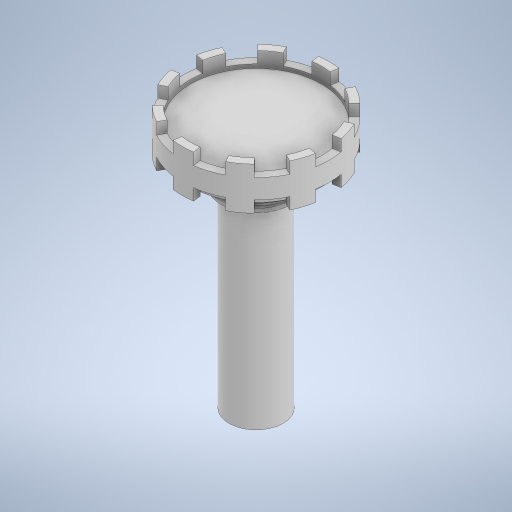
# Autodesk Inventor part: 另屋1 base
Saved by Autodesk Inventor 2024 (Build 280153000, 153)
## iProperties
Created: 2024-05-24
Part Number: 另屋1 base
Material: 一般
Document SubType Name: Modeling
Designer: User
Density: 1 g/cm^3
Appearance: 預設
Author: User
Autodesk Inventor part; units mm, degrees
ref_plane "YZ Plane" through (0, 0, 0) normal (1, 0, 0) x (0, 1, 0)
ref_plane "XZ Plane" through (0, 0, 0) normal (0, 1, 0) x (-1, 0, 0)
sketch "草圖1" plane through (0, 0, 0) normal (0, 1, 0) x (-1, 0, 0)
  circle A0 centre (0, 0) radius 19
  circle A1 centre (0, 0) radius 17
  dimension "d0" = 38
  dimension "d1" = 34
  constraints: 2 centre point, 2 coincident
  measures "d0" diameter of A0
  measures "d1" diameter of A1
extrude "擠出1" add sketch "草圖1" along normal blind 4 contours A1
extrude "擠出2" add sketch "草圖1" along normal blind 5
sketch "草圖2" plane through (0, 5, 0) normal (0, 1, 0) x (1, 0, 0)
  circle A0 centre (0, 0) radius 19
  circle A1 centre (0, 0) radius 17
  line L0 (0, 0) -> (2.6443, 18.8151)
  line L1 (0, 0) -> (-2.6443, 18.8151)
  line L2 (0, 0) -> (0, 13.9277)
  line L3 (0, 0) -> (-8.92, 16.776)
  line L4 (0, 0) -> (-13.1985, 13.6675)
  line L5 (0, 0) -> (-17.0771, 8.3291)
  line L6 (0, 0) -> (-18.7113, 3.2993)
  line L7 (0, 0) -> (-18.7113, -3.2993)
  line L8 (0, 0) -> (-17.0771, -8.3291)
  line L9 (0, 0) -> (-13.1985, -13.6675)
  line L10 (0, 0) -> (-8.92, -16.776)
  line L11 (0, 0) -> (-2.6443, -18.8151)
  line L12 (0, 0) -> (2.6443, -18.8151)
  line L13 (0, 0) -> (8.92, -16.776)
  line L14 (0, 0) -> (13.1985, -13.6675)
  line L15 (0, 0) -> (17.0771, -8.3291)
  line L16 (0, 0) -> (18.7113, -3.2993)
  line L17 (0, 0) -> (18.7113, 3.2993)
  line L18 (0, 0) -> (17.0771, 8.3291)
  line L19 (0, 0) -> (13.1985, 13.6675)
  line L20 (0, 0) -> (8.92, 16.776)
  point P0 (15.2795, 7.4523)
  point P1 (16.7417, 2.952)
  point P2 (16.7417, -2.952)
  point P3 (15.2795, -7.4523)
  point P4 (11.8092, -12.2288)
  point P5 (7.981, -15.0101)
  point P6 (2.3659, -16.8346)
  point P7 (-2.3659, -16.8346)
  point P8 (-7.981, -15.0101)
  point P9 (-11.8092, -12.2288)
  point P10 (-15.2795, -7.4523)
  point P11 (-16.7417, -2.952)
  point P12 (-16.7417, 2.952)
  point P13 (-15.2795, 7.4523)
  point P14 (-11.8092, 12.2288)
  point P15 (-7.981, 15.0101)
  point P16 (7.981, 15.0101)
  point P17 (11.8092, 12.2288)
  point P18 (-2.3659, 16.8346)
  point P19 (2.3659, 16.8346)
  dimension "d6" = 8
  dimension "d7" = 8
  dimension "d10" = 360
  constraints: 42 end point, 4 coincident, 2 centre point, 2 point on circle, 1 vertical, 49 other
  measures "d6" angle of L2 L0
  measures "d7" angle of L1 L2
extrude "擠出3" add sketch "草圖2" along normal blind 3 contours L17 A1 L18 A0 | A0 L15 A1 L16 | L19 A1 L20 A0 | A0 L13 A1 L14 | A1 L1 A0 L0 | A1 L4 A0 L3 | A1 L6 A0 L5 | A1 L8 A0 L7 | A1 L10 A0 L9 | A1 L12 A0 L11
ref_plane "工作平面1" through (0, 2.5, 0) normal (0, 1, 0) x (1, 0, 0)
mirror "鏡射1" about plane through (0, 2.5, 0) normal (0, 1, 0) of "擠出3"
sketch "草圖3" plane through (0, 0, 0) normal (0, -1, 0) x (1, 0, 0)
  circle A0 centre (0, 0) radius 17 projected
  circle A1 centre (0, 0) radius 17
  constraints: 1 centre point, 1 coincident
extrude "擠出4" add sketch "草圖3" along normal blind 2
sketch "草圖4" plane through (0, -2, 0) normal (0, -1, 0) x (1, 0, 0)
  circle A0 centre (0, 0) radius 15
  dimension "d16" = 30
  constraints: 1 centre point, 1 coincident
  measures "d16" diameter of A0
extrude "擠出5" add sketch "草圖4" along normal blind 2
sketch "草圖5" plane through (0, -4, 0) normal (0, -1, 0) x (1, 0, 0)
  circle A0 centre (0, 0) radius 13
  dimension "d19" = 26
  constraints: 1 centre point, 1 coincident
  measures "d19" diameter of A0
extrude "擠出6" add sketch "草圖5" along normal blind 2
sketch "草圖6" plane through (0, -6, 0) normal (0, -1, 0) x (1, 0, 0)
  circle A0 centre (0, 0) radius 11
  dimension "d22" = 22
  constraints: 1 centre point, 1 coincident
  measures "d22" diameter of A0
extrude "擠出7" add sketch "草圖6" along normal blind 2
sketch "草圖7" plane through (0, -8, 0) normal (0, -1, 0) x (1, 0, 0)
  circle A0 centre (0, 0) radius 9
  dimension "d25" = 18
  constraints: 1 centre point, 1 coincident
  measures "d25" diameter of A0
extrude "擠出8" add sketch "草圖7" along normal blind 2
fillet "圓角1" radius 1 8 edges at (-13.7533, -2, 9.9923) (-15, -2, 0) (-15, -4, 0) (-13, -4, 0) (-13, -6, 0) (-11, -6, 0) (-11, -8, 0) (-9, -8, 0)
sketch "草圖8" plane through (0, -10, 0) normal (0, -1, 0) x (1, 0, 0)
  circle A0 centre (0, 0) radius 7
  dimension "d29" = 14
  constraints: 1 centre point, 1 coincident
  measures "d29" diameter of A0
extrude "擠出9" add sketch "草圖8" along normal blind 50
